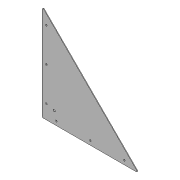
# Autodesk Inventor part: Display_CCM_Mount_Top
Saved by Autodesk Inventor 2020 (Build 240168000, 168)
## iProperties
Created: 2021-07-12
Part Number: Display_CCM_Mount_Top
Material: 一般
Document SubType Name: Sheet Metal
Designer: magnarecta
Density: 1 g/cm^3
Sheet Metal Rule: Default_mm
Appearance: 既定
Author: magnarecta
Autodesk Inventor part; units mm, degrees
ref_plane "YZ Plane" through (0, 0, 0) normal (1, 0, 0) x (0, 1, 0)
ref_plane "XZ Plane" through (0, 0, 0) normal (0, 1, 0) x (-1, 0, 0)
ref_plane "XY Plane" through (0, 0, 0) normal (0, 0, 1) x (1, 0, 0)
sketch "スケッチ1" plane through (0, 0, 0) normal (0, 0, 1) x (1, 0, 0)
  line L0 (0, 0) -> (239.9998, 0)
  line L1 (239.9998, 0) -> (239.9998, 239.9998)
  line L2 (239.9998, 239.9998) -> (0, 239.9998)
  line L3 (0, 239.9998) -> (0, 0)
  line L4 (0, 239.9998) -> (239.9998, 0)
  line L5 (-178.706, 178.706) -> (151.9787, -151.9787)
  dimension "d16" = 45
  dimension "d17" = 169.7055
  measures "d16" angle of L4 L0
  measures "d17" distance between parallel lines of L4 L5
extrude "プレート1" add sketch "スケッチ1" along normal blind 1.5 contours L3 L4 L0
sketch "スケッチ2" plane through (0, 0, 1.5) normal (0, 0, 1) x (1, 0, 0)
  line L0 (90, 33.5) -> (110, 33.5)
  line L1 (110, 33.5) -> (110, 86.5)
  line L2 (110, 86.5) -> (90, 86.5)
  line L3 (90, 86.5) -> (90, 33.5)
  line L4 (90, 33.5) -> (110, 86.5) construction
  line L5 (110, 33.5) -> (90, 86.5) construction
  line L6 (239.9998, 0) -> (0, 0) projected
  line L7 (0, 0) -> (0, 239.9998) projected
  line L8 (134, 30) -> (66, 30)
  line L9 (66, 30) -> (66, 90)
  line L10 (66, 90) -> (134, 90)
  line L11 (134, 90) -> (134, 30)
  line L12 (134, 30) -> (66, 90) construction
  line L13 (66, 30) -> (134, 90) construction
  point P0 (100, 60)
  dimension "d3" = 20
  dimension "d4" = 53
  dimension "d5" = 60
  dimension "d6" = 100
  dimension "d14" = 60
  dimension "d15" = 68
  constraints: 24 end point, 4 midpoint, 4 parallel, 2 horizontal, 2 perpendicular
  measures "d3" distance of L1.end L2.end
  measures "d4" distance of L0.end L1.end
  measures "d5" distance from line of point (100, 60) L6
  measures "d6" distance from line of point (100, 60) L7
  measures "d14" distance of L8.end L9.end
  measures "d15" distance of L8.start L8.end
hole "穴1" at (90, 33.5, 1.5) at (110, 33.5, 1.5) at (90, 86.5, 1.5) at (110, 86.5, 1.5) at (66, 30, 1.5) at (134, 30, 1.5) at (66, 90, 1.5) direction (0, 0, -1) diameter 5.2 depth 1.5 tip angle 118
fillet "フィレット1" radius 2 3 edges at (0, 239.9998, 0.75) (0, 0, 0.75) (239.9998, 0, 0.75)
sketch "スケッチ3" plane through (0, 0, 1.5) normal (0, 0, 1) x (1, 0, 0)
  circle A0 centre (66, 90) radius 2.6 projected
  line L0 (0, 2) -> (0, 235.1714) projected
  point P0 (0, 0)
  point P1 (90, 117)
  point P2 (80, 117)
  dimension "d19" = 10
  dimension "d20" = 27
  dimension "d21" = 80
  constraints: 1 horizontal alignment
  measures "d19" distance of point (80, 117) point (90, 117)
  measures "d20" vertical distance of A0.centre point (80, 117)
  measures "d21" distance from line of L0 point (80, 117)
hole "穴2" at (90, 117, 1.5) at (80, 117, 1.5) direction (0, 0, -1) diameter 3.242 depth 11.8 tip angle 118 thread size "M4x0.7" class "6H" standard "ISO Metric profile"
sketch "スケッチ4" plane through (0, 0, 1.5) normal (0, 0, 1) x (1, 0, 0)
  circle A0 centre (90, 117) radius 1.621 projected
  circle A1 centre (80, 117) radius 1.621 projected
  arc A2 (235.1714, 0) -> (236.5856, 3.4142) centre (235.1714, 2) ccw projected
  line L0 (3.4142, 236.5856) -> (236.5856, 3.4142) projected
  arc A3 (3.4142, 236.5856) -> (0, 235.1714) centre (2, 235.1714) ccw projected
  line L1 (0, 2) -> (0, 235.1714) projected
  arc A4 (0, 2) -> (2, 0) centre (2, 2) ccw projected
  line L2 (235.1714, 0) -> (2, 0) projected
  circle A5 centre (134, 30) radius 2.6 projected
  circle A6 centre (110, 86.5) radius 2.6 projected
  circle A7 centre (110, 33.5) radius 2.6 projected
  circle A8 centre (90, 33.5) radius 2.6 projected
  circle A9 centre (90, 86.5) radius 2.6 projected
  circle A10 centre (66, 30) radius 2.6 projected
  circle A11 centre (66, 90) radius 2.6 projected
  line L3 (10, 10) -> (10, 215.8577)
  line L4 (10, 215.8577) -> (215.8577, 10)
  line L5 (215.8577, 10) -> (10, 10)
  point P0 (0, 0)
  point P1 (205, 10)
  point P2 (35, 10)
  point P3 (10, 35)
  point P4 (10, 205)
  point P5 (120, 10)
  point P6 (10, 120)
  dimension "d29" = 10
  dimension "d30" = 25
  dimension "d31" = 25
  dimension "d32" = 170
  dimension "d33" = 170
  dimension "d34" = 85
  dimension "d35" = 85
  constraints: 6 end point, 6 point on line, 1 coincident, 2 other
  measures "d29" distance between parallel lines of L2 L5
  measures "d30" horizontal distance of point (10, 35) point (35, 10)
  measures "d31" distance of point (10, 10) point (10, 35)
  measures "d32" distance of point (35, 10) point (205, 10)
  measures "d33" distance of point (10, 35) point (10, 205)
  measures "d34" distance of point (10, 120) point (10, 35)
  measures "d35" distance of point (35, 10) point (120, 10)
hole "穴3" at (205, 10, 1.5) at (35, 10, 1.5) at (10, 35, 1.5) at (10, 205, 1.5) at (120, 10, 1.5) at (10, 120, 1.5) direction (0, 0, -1) diameter 4.2 depth 1.5 tip angle 118
sketch "スケッチ6" plane through (0, 0, 1.5) normal (0, 0, 1) x (1, 0, 0)
  circle A0 centre (120, 10) radius 2.1 projected
  circle A1 centre (10, 35) radius 2.1 projected
  circle A2 centre (205, 10) radius 2.1 projected
  circle A3 centre (35, 10) radius 2.1 projected
  circle A4 centre (10, 205) radius 2.1 projected
  circle A5 centre (10, 120) radius 2.1 projected
  circle A6 centre (90, 117) radius 1.621 projected
  circle A7 centre (80, 117) radius 1.621 projected
  arc A8 (235.1714, 0) -> (236.5856, 3.4142) centre (235.1714, 2) ccw projected
  line L0 (3.4142, 236.5856) -> (236.5856, 3.4142) projected
  arc A9 (3.4142, 236.5856) -> (0, 235.1714) centre (2, 235.1714) ccw projected
  line L1 (0, 2) -> (0, 235.1714) projected
  arc A10 (0, 2) -> (2, 0) centre (2, 2) ccw projected
  line L2 (235.1714, 0) -> (2, 0) projected
  circle A11 centre (134, 30) radius 2.6 projected
  circle A12 centre (110, 86.5) radius 2.6 projected
  circle A13 centre (110, 33.5) radius 2.6 projected
  circle A14 centre (90, 33.5) radius 2.6 projected
  circle A15 centre (90, 86.5) radius 2.6 projected
  circle A16 centre (66, 30) radius 2.6 projected
  circle A17 centre (66, 90) radius 2.6 projected
  line L3 (20, 20) -> (20, 191.7155)
  line L4 (20, 191.7155) -> (191.7155, 20)
  line L5 (191.7155, 20) -> (20, 20)
  point P0 (0, 0)
  point P1 (30, 30)
  dimension "d46" = 20
  dimension "d47" = 10
  dimension "d48" = 10
  constraints: 6 end point, 2 other
  measures "d46" distance between parallel lines of L2 L5
  measures "d47" distance from line of L3 point (30, 30)
  measures "d48" distance from line of L5 point (30, 30)
hole "穴4" at (30, 30, 1.5) direction (0, 0, -1) diameter 5.2 depth 1.5 tip angle 118
sketch "スケッチ7" plane through (0, 0, 1.5) normal (0, 0, 1) x (1, 0, 0)
  circle A0 centre (30, 30) radius 2.6 projected
  circle A1 centre (120, 10) radius 2.1 projected
  circle A2 centre (10, 35) radius 2.1 projected
  circle A3 centre (205, 10) radius 2.1 projected
  circle A4 centre (35, 10) radius 2.1 projected
  circle A5 centre (10, 205) radius 2.1 projected
  circle A6 centre (10, 120) radius 2.1 projected
  circle A7 centre (90, 117) radius 1.621 projected
  circle A8 centre (80, 117) radius 1.621 projected
  arc A9 (235.1714, 0) -> (236.5856, 3.4142) centre (235.1714, 2) ccw projected
  line L0 (3.4142, 236.5856) -> (236.5856, 3.4142) projected
  arc A10 (3.4142, 236.5856) -> (0, 235.1714) centre (2, 235.1714) ccw projected
  line L1 (0, 2) -> (0, 235.1714) projected
  arc A11 (0, 2) -> (2, 0) centre (2, 2) ccw projected
  line L2 (235.1714, 0) -> (2, 0) projected
  circle A12 centre (134, 30) radius 2.6 projected
  circle A13 centre (110, 86.5) radius 2.6 projected
  circle A14 centre (110, 33.5) radius 2.6 projected
  circle A15 centre (90, 33.5) radius 2.6 projected
  circle A16 centre (90, 86.5) radius 2.6 projected
  circle A17 centre (66, 30) radius 2.6 projected
  circle A18 centre (66, 90) radius 2.6 projected
  point P0 (0, 0)
extrude "押し出し2" add sketch "スケッチ7" against normal up to surface (1.5 mm away) contours A7 | A8 | A12 | A13 | A14 | A15 | A16 | A17 | A18
equation "\"d12\" = Thickness"
equation "\"d41\" = Thickness"
equation "\"d54\" = Thickness"
equation "\"d2\" = Thickness"
equation "\"BendRadius\" = Thickness"
equation "\"BendReliefWidth\" = Thickness"
equation "\"BendReliefDepth\" = 0.5 * Thickness"
equation "\"CornerReliefSize\" = 4 * Thickness"
equation "\"MinimumRemnant\" = 2 * Thickness"
equation "\"TransitionRadius\" = BendRadius"
equation "\"JacobiRadiusSize\" = BendRadius"
equation "\"GapSize\" = Thickness"
equation "\"Thickness\" = 1.5"
